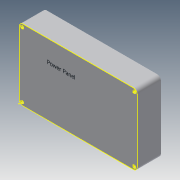
# Autodesk Inventor part: power panel
Saved by Autodesk Inventor 2014 (Build 180170000, 170)
## iProperties
Created: 2016-01-12
Part Number: power panel
Material: Generic
Document SubType Name: Modeling
Designer: Paul
Density: 1 g/cm^3
Appearance: Default
Author: Paul
Autodesk Inventor part; units mm, degrees
ref_plane "YZ Plane" through (0, 0, 0) normal (1, 0, 0) x (0, 1, 0)
ref_plane "XZ Plane" through (0, 0, 0) normal (0, 1, 0) x (-1, 0, 0)
ref_plane "XY Plane" through (0, 0, 0) normal (0, 0, 1) x (1, 0, 0)
sketch "Sketch1" plane through (0, 0, 0) normal (0, 0, 1) x (1, 0, 0)
  line L0 (0, 0) -> (190.5, 0)
  line L1 (190.5, 0) -> (190.5, 114.3)
  line L2 (190.5, 114.3) -> (0, 114.3)
  line L3 (0, 114.3) -> (0, 0)
  dimension "d0" = 190.5
  dimension "d1" = 114.3
  constraints: 8 end point, 2 parallel, 1 coincident, 1 horizontal, 1 perpendicular
  measures "d0" distance of L2.end L1.end
  measures "d1" distance of L1.end L0.end
extrude "Extrusion1" add sketch "Sketch1" along normal blind 38.1
fillet "Fillet1" radius 6.35 4 edges at (190.5, 114.3, 19.05) (190.5, 0, 19.05) (0, 114.3, 19.05) (0, 0, 19.05)
sketch "Sketch2" plane through (0, 0, 38.1) normal (0, 0, 1) x (1, 0, 0)
  line L0 (6.35, 0) -> (184.15, 0) projected
  line L1 (0, 107.95) -> (0, 6.35) projected
  line L2 (4.7625, 109.5375) -> (4.7625, 4.7625)
  line L3 (4.7625, 4.7625) -> (185.7375, 4.7625)
  point P0 (0, 0)
  point P1 (185.7375, 109.5375)
  point P2 (4.7625, 57.15)
  point P3 (0, 57.15)
  point P4 (95.25, 4.7625)
  point P5 (95.25, 0)
  dimension "d5" = 180.975
  dimension "d6" = 104.775
  dimension "d7" = 180.975
  constraints: 4 end point, 4 midpoint, 1 horizontal alignment, 1 parallel, 1 perpendicular, 1 vertical alignment
  measures "d5" distance of point (185.738, 109.538) L2.start
  measures "d6" distance of L2.start L2.end
  measures "d7" distance of L3.end L2.end
hole "Hole1" at (4.7625, 109.5375, 38.1) at (4.7625, 4.7625, 38.1) at (185.7375, 4.7625, 38.1) at (185.7375, 109.5375, 38.1) direction (0, 0, -1) diameter 4.7625 depth 25.4 tip angle 118
sketch "Sketch3" plane through (0, 0, 38.1) normal (0, 0, 1) x (1, 0, 0)
  circle A0 centre (185.7375, 4.7625) radius 2.3813 projected
  circle A1 centre (4.7625, 109.5375) radius 2.3813 projected
  circle A2 centre (4.7625, 4.7625) radius 2.3813 projected
  circle A3 centre (185.7375, 109.5375) radius 2.3813 projected
  arc A4 (0, 6.35) -> (6.35, 0) centre (6.35, 6.35) ccw projected
  line L0 (6.35, 0) -> (184.15, 0) projected
  arc A5 (184.15, 0) -> (190.5, 6.35) centre (184.15, 6.35) ccw projected
  line L1 (190.5, 6.35) -> (190.5, 107.95) projected
  arc A6 (190.5, 107.95) -> (184.15, 114.3) centre (184.15, 107.95) ccw projected
  line L2 (184.15, 114.3) -> (6.35, 114.3) projected
  arc A7 (6.35, 114.3) -> (0, 107.95) centre (6.35, 107.95) ccw projected
  line L3 (0, 107.95) -> (0, 6.35) projected
  line L4 (45.0816, 84.7015) -> (137.1941, 84.7015) construction
  line L5 (137.1941, 84.7015) -> (137.1941, 62.4958) construction
  line L6 (137.1941, 62.4958) -> (45.0816, 62.4958) construction
  line L7 (45.0816, 62.4958) -> (45.0816, 84.7015) construction
  point P0 (0, 0)
  constraints: 2 other
body "Solid1"
